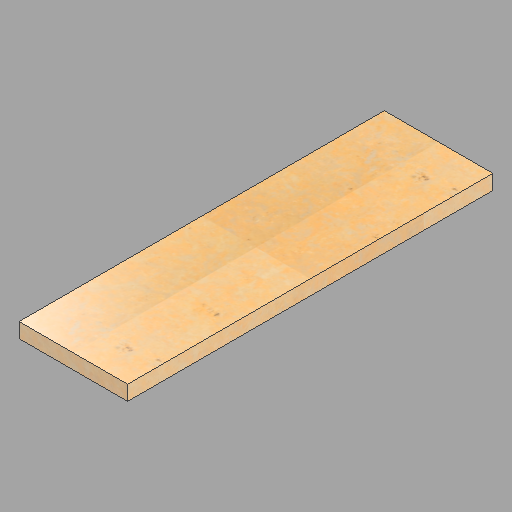
# Autodesk Inventor part: B - Cap - 1
Saved by Autodesk Inventor 2022.2 (Build 262287010, 287A)
## iProperties
RuleStatus: InUse
Created: 2022-03-23
Part Number: B - Cap - 1
Material: Granite, Cut, Polished
Document SubType Name: Modeling
Designer: awelt
Mass: 215573 g
Surface Area: 25329 cm^2
Volume: 79841.9 cm^3
Density: 2.7 g/cm^3
Appearance: Amber Select
AfterDocSave0: Convert in3 volume to ft3
in3 to ft3: 2.82
TEST: 2.82
Author: awelt
Autodesk Inventor part; units mm, degrees
ref_plane "YZ Plane" through (0, 0, 0) normal (1, 0, 0) x (0, 1, 0)
ref_plane "XZ Plane" through (0, 0, 0) normal (0, 1, 0) x (-1, 0, 0)
ref_plane "XY Plane" through (0, 0, 0) normal (0, 0, 1) x (1, 0, 0)
sketch "Sketch1" plane through (0, 0, 0) normal (0, 1, 0) x (-1, 0, 0)
  line L0 (279.4, 939.8) -> (-279.4, 939.8)
  line L1 (-279.4, 939.8) -> (-279.4, -939.8)
  line L2 (-279.4, -939.8) -> (279.4, -939.8)
  line L3 (279.4, -939.8) -> (279.4, 939.8)
  line L4 (279.4, 939.8) -> (-279.4, -939.8) construction
  line L5 (-279.4, 939.8) -> (279.4, -939.8) construction
  line L6 (269.875, 930.275) -> (-269.875, 930.275)
  line L7 (-269.875, 930.275) -> (-269.875, -930.275)
  line L8 (-269.875, -930.275) -> (269.875, -930.275)
  line L9 (269.875, -930.275) -> (269.875, 930.275)
  line L10 (263.525, 923.925) -> (-263.525, 923.925)
  line L11 (-263.525, 923.925) -> (-263.525, -923.925)
  line L12 (-263.525, -923.925) -> (263.525, -923.925)
  line L13 (263.525, -923.925) -> (263.525, 923.925)
  point P0 (0, 0)
  dimension "d2" = 558.8
  dimension "d3" = 1879.6
  dimension "d4" = 9.525
  dimension "d5" = 6.35
  constraints: 28 end point, 6 parallel, 3 perpendicular, 2 midpoint, 1 horizontal, 6 other
  measures "d2" distance of L2.end L1.end
  measures "d3" distance of L1.end L0.end
  measures "d4" distance between parallel lines of L3 L9
  measures "d5" distance between parallel lines of L9 L13
extrude "Extrusion1" add sketch "Sketch1" along normal blind 76.2 contours L3 L2 L1 L0 | L9 L8 L7 L6 | L13 L12 L11 L10
extrude "Extrusion3" cut sketch "Sketch1" along normal blind 6.35 contours L9 L8 L7 L6
body "Solid1"
